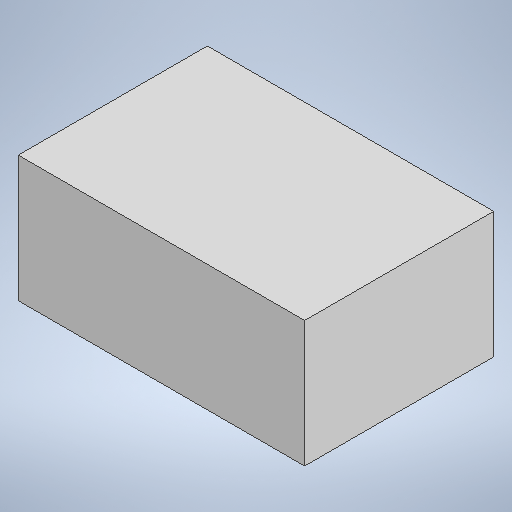
# Autodesk Inventor part: Custom.Motor.Caps
Saved by Autodesk Inventor 2025.1 (Build 291241020, 241B)
## iProperties
Created: 2024-10-10
Part Number: Custom.Motor.Caps
Material: Generic
Document SubType Name: Modeling
Designer: raulh
Density: 1 g/cm^3
Appearance: Default
Author: raulh
Autodesk Inventor part; units mm, degrees
ref_plane "YZ Plane" through (0, 0, 0) normal (1, 0, 0) x (0, 1, 0)
ref_plane "XZ Plane" through (0, 0, 0) normal (0, 1, 0) x (-1, 0, 0)
ref_plane "XY Plane" through (0, 0, 0) normal (0, 0, 1) x (1, 0, 0)
sketch "Sketch1" plane through (0, 0, 0) normal (0, 1, 0) x (-1, 0, 0)
  line L0 (29.5105, 21.6537) -> (-28.1983, 21.6537)
  line L1 (-28.1983, 21.6537) -> (-28.1983, -16.4463)
  line L2 (-28.1983, -16.4463) -> (29.5105, -16.4463)
  line L3 (29.5105, -16.4463) -> (29.5105, 21.6537)
  point P0 (0, 0)
  dimension "d0" = 57.7088
  dimension "d1" = 38.1
  constraints: 8 end point, 2 parallel, 1 horizontal, 1 perpendicular
  measures "d0" distance of L1.end L2.end
  measures "d1" distance of L0.end L1.end
extrude "Extrusion1" add sketch "Sketch1" along normal blind 25.4
body "Solid1"
